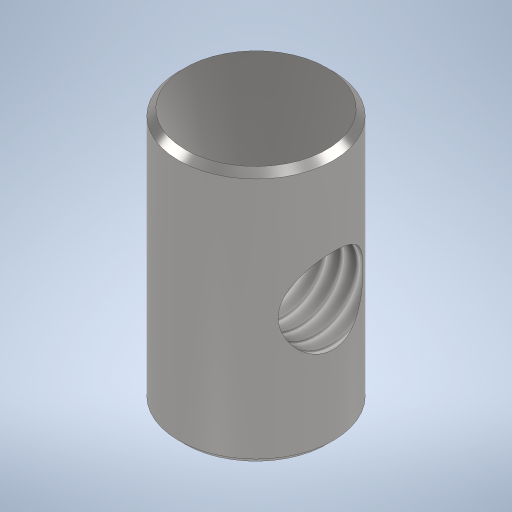
# Autodesk Inventor part: Pasador roscado DC
Saved by Autodesk Inventor 2024.2 (Build 282272000, 272)
## iProperties
Created: 2026-07-16
Part Number: Pasador roscado DC
Material: Steel, Carbon
Document SubType Name: Modeling
Designer: ja.restrepo1
Density: 7.85 g/cm^3
Appearance: Semi-Polished
Author: ja.restrepo1
Autodesk Inventor part; units mm, degrees
ref_plane "XZ Plane" through (0, 0, 0) normal (0, 1, 0) x (-1, 0, 0)
ref_plane "XY Plane" through (0, 0, 0) normal (0, 0, 1) x (1, 0, 0)
sketch "Sketch1" plane through (0, 0, 0) normal (1, 0, 0) x (0, 1, 0)
  line L0 (9.5, 6.05) -> (-9.5, 6.05)
  line L1 (-10, 5.55) -> (-10, 0)
  line L2 (-10, 0) -> (10, 0)
  line L3 (10, 0) -> (10, 5.55)
  line L4 (9.5, 6.05) -> (10, 5.55)
  line L5 (-9.5, 6.05) -> (-10, 5.55)
  point P0 (0, 0)
  point P1 (10, 6.05)
  point P2 (-10, 6.05)
  point P3 (0, 0)
  dimension "d0" = 20
  dimension "d1" = 6.05
  dimension "d2" = 0.5
  dimension "d3" = 0.5
  dimension "d4" = 0.5
  dimension "d5" = 0.5
  constraints: 12 end point, 4 point on line, 2 coincident, 2 parallel, 1 horizontal, 1 midpoint, 1 perpendicular
  measures "d0" distance of L2.end L1.end
  measures "d1" distance of L1.end point (-10, 6.05)
  measures "d2" distance of L0.start point (10, 6.05)
  measures "d3" distance of L3.end point (10, 6.05)
  measures "d4" distance of L0.end point (-10, 6.05)
  measures "d5" distance of L1.start point (-10, 6.05)
revolve "Pasador Ø12" add sketch "Sketch1" angle 360 about axis through (0, -10, 0) along (0, 1, 0)
ref_plane "Work Plane1" through (6.1, 0, 0) normal (1, 0, 0) x (0, 1, 0)
sketch "Sketch2" plane through (6.1, 0, 0) normal (1, 0, 0) x (0, 1, 0)
  point P0 (0, 0)
  point P1 (0, 0)
  constraints: 1 coincident
hole "M8" at (6.1, 0, 0) at (6.1, 0, 0) direction (-1, 0, 0) diameter 6.647 end through all thread size "M8x1.25" class "6H" standard "ANSI Metric M Profile"
equation "\"d3\" = d2"
equation "\"d4\" = d2"
equation "\"d5\" = d4"
body "Solid1"
